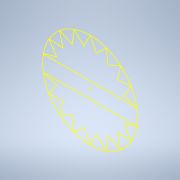
# Autodesk Inventor part: PotAttachmentB10R
Saved by Autodesk Inventor 2022 (Build 260153000, 153)
## iProperties
Created: 2021-12-04
Part Number: PotAttachmentB10R
Material: Generic
Document SubType Name: Modeling
Designer: teh18
Density: 1 g/cm^3
Appearance: Default
Author: teh18
Autodesk Inventor part; units mm, degrees
ref_plane "YZ Plane" through (0, 0, 0) normal (1, 0, 0) x (0, 1, 0)
ref_plane "XZ Plane" through (0, 0, 0) normal (0, 1, 0) x (-1, 0, 0)
ref_plane "XY Plane" through (0, 0, 0) normal (0, 0, 1) x (1, 0, 0)
ref_plane "Work Plane1" through (-2.5858, -0.1842, 12) normal (0, 0, 1) x (1, 0, 0)
sketch "Sketch1" plane through (0, 0, 0) normal (0, 0, 1) x (1, 0, 0)
  line L0 (-1.7235, 1.3627) -> (-1.9283, 2.2145) projected
  arc A0 (-1.9283, 2.2145) -> (-2.598, 1.4164) centre (0.0001, -0.0836) ccw projected
  line L1 (-2.598, 1.4164) -> (-1.7235, 1.3627) projected
  line L2 (-1.1249, 1.865) -> (-1.026, 2.7355) projected
  arc A1 (-1.026, 2.7355) -> (-1.9283, 2.2145) centre (0.0001, -0.0836) ccw projected
  line L3 (-1.9283, 2.2145) -> (-1.1249, 1.865) projected
  line L4 (-0.3906, 2.1322) -> (0.0001, 2.9164) projected
  arc A2 (0.0001, 2.9164) -> (-1.026, 2.7355) centre (0.0001, -0.0836) ccw projected
  line L5 (-1.026, 2.7355) -> (-0.3906, 2.1322) projected
  line L6 (0.3908, 2.1322) -> (1.0261, 2.7355) projected
  arc A3 (1.0261, 2.7355) -> (0.0001, 2.9164) centre (0.0001, -0.0836) ccw projected
  line L7 (0.0001, 2.9164) -> (0.3908, 2.1322) projected
  line L8 (1.0261, 2.7355) -> (1.1251, 1.865) projected
  line L9 (1.1251, 1.865) -> (1.9284, 2.2145) projected
  arc A4 (1.9284, 2.2145) -> (1.0261, 2.7355) centre (0.0001, -0.0836) ccw projected
  line L10 (1.9284, 2.2145) -> (1.7237, 1.3627) projected
  line L11 (1.7237, 1.3627) -> (2.5982, 1.4164) projected
  arc A5 (2.5982, 1.4164) -> (1.9284, 2.2145) centre (0.0001, -0.0836) ccw projected
  line L12 (2.5982, 1.4164) -> (2.1144, 0.6859) projected
  line L13 (2.1144, 0.6859) -> (2.9545, 0.4373) projected
  arc A6 (2.9545, 0.4373) -> (2.5982, 1.4164) centre (0.0001, -0.0836) ccw projected
  line L14 (-2.9543, -0.6046) -> (-2.926, -0.5836) projected
  line L15 (-2.926, -0.5836) -> (2.9262, -0.5836) projected
  line L16 (2.9262, -0.5836) -> (2.9545, -0.6046) projected
  arc A7 (2.9545, -0.6046) -> (2.9545, 0.4373) centre (0.0001, -0.0836) ccw projected
  line L17 (2.9545, 0.4373) -> (2.9262, 0.4164) projected
  line L18 (2.9262, 0.4164) -> (-2.926, 0.4164) projected
  line L19 (-2.926, 0.4164) -> (-2.9543, 0.4373) projected
  arc A8 (-2.9543, 0.4373) -> (-2.9543, -0.6046) centre (0.0001, -0.0836) ccw projected
  line L20 (2.9545, -0.6046) -> (2.1144, -0.8532) projected
  line L21 (2.1144, -0.8532) -> (2.5982, -1.5836) projected
  arc A9 (2.5982, -1.5836) -> (2.9545, -0.6046) centre (0.0001, -0.0836) ccw projected
  line L22 (2.5982, -1.5836) -> (1.7237, -1.5299) projected
  line L23 (1.7237, -1.5299) -> (1.9284, -2.3817) projected
  arc A10 (1.9284, -2.3817) -> (2.5982, -1.5836) centre (0.0001, -0.0836) ccw projected
  line L24 (1.1251, -2.0322) -> (1.0261, -2.9027) projected
  arc A11 (1.0261, -2.9027) -> (1.9284, -2.3817) centre (0.0001, -0.0836) ccw projected
  line L25 (1.9284, -2.3817) -> (1.1251, -2.0322) projected
  line L26 (0.3908, -2.2994) -> (0.0001, -3.0836) projected
  arc A12 (0.0001, -3.0836) -> (1.0261, -2.9027) centre (0.0001, -0.0836) ccw projected
  line L27 (1.0261, -2.9027) -> (0.3908, -2.2994) projected
  line L28 (-0.3906, -2.2994) -> (-1.026, -2.9027) projected
  arc A13 (-1.026, -2.9027) -> (0.0001, -3.0836) centre (0.0001, -0.0836) ccw projected
  line L29 (0.0001, -3.0836) -> (-0.3906, -2.2994) projected
  line L30 (-1.1249, -2.0322) -> (-1.9283, -2.3817) projected
  arc A14 (-1.9283, -2.3817) -> (-1.026, -2.9027) centre (0.0001, -0.0836) ccw projected
  line L31 (-1.026, -2.9027) -> (-1.1249, -2.0322) projected
  line L32 (-1.7235, -1.5299) -> (-2.598, -1.5836) projected
  arc A15 (-2.598, -1.5836) -> (-1.9283, -2.3817) centre (0.0001, -0.0836) ccw projected
  line L33 (-1.9283, -2.3817) -> (-1.7235, -1.5299) projected
  line L34 (-2.598, -1.5836) -> (-2.1142, -0.8532) projected
  line L35 (-2.1142, -0.8532) -> (-2.9543, -0.6046) projected
  arc A16 (-2.9543, -0.6046) -> (-2.598, -1.5836) centre (0.0001, -0.0836) ccw projected
  line L36 (-2.9543, 0.4373) -> (-2.1142, 0.6859) projected
  line L37 (-2.1142, 0.6859) -> (-2.598, 1.4164) projected
  arc A17 (-2.598, 1.4164) -> (-2.9543, 0.4373) centre (0.0001, -0.0836) ccw projected
  circle A18 centre (0.0001, -0.0836) radius 3.5
  point P0 (0, 0)
  dimension "d2" = 7
  constraints: 1 centre point, 1 coincident
  measures "d2" diameter of A18
extrude "Extrusion1" add sketch "Sketch1" along normal up to surface (12 mm away) contours L1 A0 L0 | A1 L2 L3 | L37 L36 A17 | A2 L4 L5 | L19 L18 L17 A7 L16 L15 L14 A8 | A3 L6 L7 | L35 L34 A16 | A4 L9 L8 | L32 L33 A15 | A5 L11 L10 | L13 L12 A6 | L30 L31 A14 | A9 L21 L20 | L28 L29 A13 | A10 L23 L22 | L26 L27 A12 | A11 L24 L25 | A18
sketch "Sketch2" plane through (0.0001, -0.0836, 12) normal (0, 0, 1) x (1, 0, 0)
  circle A0 centre (0, 0) radius 3.5
  point P0 (-0.0001, 0.0836)
  dimension "d3" = 7
  constraints: 1 centre point
  measures "d3" diameter of A0
extrude "Extrusion2" add sketch "Sketch2" along normal blind 2
sketch "Sketch3" plane through (0.0001, -0.0836, 14) normal (0, 0, 1) x (1, 0, 0)
  circle A0 centre (0, 0) radius 3.5 projected
  line L0 (0, -4.6547) -> (-1, -2.9226)
  line L1 (-1, -2.9226) -> (1, -2.9226)
  line L2 (1, -2.9226) -> (0, -4.6547)
  line L3 (1.4642, -4.4228) -> (-0.0221, -3.0845)
  line L4 (-0.0221, -3.0845) -> (1.88, -2.4665)
  line L5 (1.88, -2.4665) -> (1.4642, -4.4228)
  line L6 (2.7851, -3.7497) -> (0.958, -2.9362)
  line L7 (0.958, -2.9362) -> (2.576, -1.7607)
  line L8 (2.576, -1.7607) -> (2.7851, -3.7497)
  line L9 (3.8333, -2.7014) -> (1.8443, -2.4924)
  line L10 (1.8443, -2.4924) -> (3.0199, -0.8743)
  line L11 (3.0199, -0.8743) -> (3.8333, -2.7014)
  line L12 (4.5063, -1.3805) -> (2.55, -1.7964)
  line L13 (2.55, -1.7964) -> (3.1681, 0.1058)
  line L14 (3.1681, 0.1058) -> (4.5063, -1.3805)
  line L15 (4.7382, 0.0837) -> (3.0062, -0.9163)
  line L16 (3.0062, -0.9163) -> (3.0062, 1.0837)
  line L17 (3.0062, 1.0837) -> (4.7382, 0.0837)
  line L18 (4.5063, 1.5479) -> (3.168, 0.0616)
  line L19 (3.168, 0.0616) -> (2.55, 1.9637)
  line L20 (2.55, 1.9637) -> (4.5063, 1.5479)
  line L21 (3.8332, 2.8688) -> (3.0198, 1.0417)
  line L22 (3.0198, 1.0417) -> (1.8442, 2.6597)
  line L23 (1.8442, 2.6597) -> (3.8332, 2.8688)
  line L24 (2.785, 3.917) -> (2.5759, 1.928)
  line L25 (2.5759, 1.928) -> (0.9579, 3.1035)
  line L26 (0.9579, 3.1035) -> (2.785, 3.917)
  line L27 (1.4641, 4.59) -> (1.8799, 2.6337)
  line L28 (1.8799, 2.6337) -> (-0.0222, 3.2518)
  line L29 (-0.0222, 3.2518) -> (1.4641, 4.59)
  line L30 (-0.0002, 4.8219) -> (0.9998, 3.0899)
  line L31 (0.9998, 3.0899) -> (-1.0002, 3.0899)
  line L32 (-1.0002, 3.0899) -> (-0.0002, 4.8219)
  line L33 (-1.4644, 4.59) -> (0.0219, 3.2517)
  line L34 (0.0219, 3.2517) -> (-1.8802, 2.6337)
  line L35 (-1.8802, 2.6337) -> (-1.4644, 4.59)
  line L36 (-2.7852, 3.9169) -> (-0.9582, 3.1035)
  line L37 (-0.9582, 3.1035) -> (-2.5762, 1.9279)
  line L38 (-2.5762, 1.9279) -> (-2.7852, 3.9169)
  line L39 (-3.8335, 2.8687) -> (-1.8444, 2.6596)
  line L40 (-1.8444, 2.6596) -> (-3.02, 1.0416)
  line L41 (-3.02, 1.0416) -> (-3.8335, 2.8687)
  line L42 (-4.5065, 1.5478) -> (-2.5502, 1.9636)
  line L43 (-2.5502, 1.9636) -> (-3.1682, 0.0615)
  line L44 (-3.1682, 0.0615) -> (-4.5065, 1.5478)
  line L45 (-4.7384, 0.0835) -> (-3.0063, 1.0835)
  line L46 (-3.0063, 1.0835) -> (-3.0063, -0.9165)
  line L47 (-3.0063, -0.9165) -> (-4.7384, 0.0835)
  line L48 (-4.5065, -1.3807) -> (-3.1682, 0.1056)
  line L49 (-3.1682, 0.1056) -> (-2.5502, -1.7965)
  line L50 (-2.5502, -1.7965) -> (-4.5065, -1.3807)
  line L51 (-3.8334, -2.7016) -> (-3.0199, -0.8745)
  line L52 (-3.0199, -0.8745) -> (-1.8444, -2.4925)
  line L53 (-1.8444, -2.4925) -> (-3.8334, -2.7016)
  line L54 (-2.7851, -3.7498) -> (-2.5761, -1.7608)
  line L55 (-2.5761, -1.7608) -> (-0.958, -2.9363)
  line L56 (-0.958, -2.9363) -> (-2.7851, -3.7498)
  line L57 (-1.4642, -4.4228) -> (-1.88, -2.4665)
  line L58 (-1.88, -2.4665) -> (0.0221, -3.0846)
  line L59 (0.0221, -3.0846) -> (-1.4642, -4.4228)
  point P0 (-0.0001, 0.0836)
  point P1 (0, -3.5)
  point P2 (1.1074, -3.3246)
  point P3 (2.1064, -2.8155)
  point P4 (2.8992, -2.0227)
  point P5 (3.4082, -1.0237)
  point P6 (3.5835, 0.0837)
  point P7 (3.4081, 1.1911)
  point P8 (2.8991, 2.1901)
  point P9 (2.1063, 2.9828)
  point P10 (1.1072, 3.4918)
  point P11 (-0.0002, 3.6672)
  point P12 (-1.1075, 3.4918)
  point P13 (-2.1065, 2.9828)
  point P14 (-2.8993, 2.1899)
  point P15 (-3.4083, 1.1909)
  point P16 (-3.5837, 0.0835)
  point P17 (-3.4083, -1.0239)
  point P18 (-2.8992, -2.0228)
  point P19 (-2.1064, -2.8156)
  point P20 (-1.1074, -3.3246)
  point P21 (0.5889, -3.6347)
  point P22 (1.7091, -3.2707)
  point P23 (2.662, -2.5783)
  point P24 (3.3543, -1.6254)
  point P25 (3.7182, -0.5052)
  point P26 (3.7182, 0.6726)
  point P27 (3.3542, 1.7928)
  point P28 (2.6619, 2.7457)
  point P29 (1.7089, 3.4379)
  point P30 (0.5888, 3.8019)
  point P31 (-0.5891, 3.8019)
  point P32 (-1.7093, 3.4379)
  point P33 (-2.6621, 2.7455)
  point P34 (-3.3544, 1.7926)
  point P35 (-3.7184, 0.6724)
  point P36 (-3.7183, -0.5054)
  point P37 (-3.3543, -1.6256)
  point P38 (-2.662, -2.5784)
  point P39 (-1.7091, -3.2707)
  point P40 (-0.5889, -3.6347)
  dimension "d6" = 2
  dimension "d9" = 360
  constraints: 120 end point, 2 vertical alignment, 1 horizontal alignment, 149 other
  measures "d6" distance of L0.end L1.end
extrude "Extrusion3" add sketch "Sketch3" against normal blind 8
body "Solid1"
